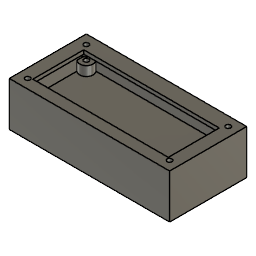
1602L_display_case (Autodesk Fusion 360 design; units mm, degrees)
Autodesk Fusion 360 part; units mm, degrees
sketch "Sketch1" plane through (0, 0, 0) normal (0, 0, 1) x (1, 0, 0)
  line L0 (0, 0) -> (80, 0)
  line L1 (80, 0) -> (80, 36)
  line L2 (80, 36) -> (0, 36)
  line L3 (0, 36) -> (0, 0)
  line L4 (-2.4, -2.4) -> (82.4, -2.4)
  line L5 (82.4, -2.4) -> (82.4, 38.4)
  line L6 (82.4, 38.4) -> (-2.4, 38.4)
  line L7 (-2.4, 38.4) -> (-2.4, -2.4)
  circle A0 centre (2.5, 33.5) radius 1.3
  circle A1 centre (2.5, 2.5) radius 1.3
  circle A2 centre (77.5, 2.5) radius 1.3
  circle A3 centre (77.5, 33.5) radius 1.3
  line L8 (4.2, 30.4) -> (75.8, 30.4)
  line L9 (75.8, 30.4) -> (75.8, 3.5)
  line L10 (75.8, 3.5) -> (4.2, 3.5)
  line L11 (4.2, 3.5) -> (4.2, 30.4)
  circle A4 centre (2.5, 33.5) radius 3.5
  circle A5 centre (77.5, 33.5) radius 3.5
  line L12 (-0.4, -0.4) -> (80.4, -0.4)
  line L13 (80.4, -0.4) -> (80.4, 36.4)
  line L14 (80.4, 36.4) -> (-0.4, 36.4)
  line L15 (-0.4, 36.4) -> (-0.4, -0.4)
  line L16 (-0.4, 6) -> (4.2, 6)
  line L17 (6, 3.5) -> (6, -0.4)
  line L18 (75.8, 6) -> (80.4, 6)
  line L19 (74, 3.5) -> (74, -0.4)
  circle A6 centre (2.5, 2.5) radius 3.5
  circle A7 centre (77.5, 2.5) radius 3.5
  point P0 (8, 33.5)
  dimension "d1" = 80
  dimension "d2" = 36
  dimension "d4" = 2.6
  dimension "d5" = 2.6
  dimension "d6" = 2.6
  dimension "d7" = 2.6
  dimension "d8" = 2.5
  dimension "d9" = 2.5
  dimension "d10" = 2.5
  dimension "d11" = 2.5
  dimension "d12" = 2.5
  dimension "d13" = 2.5
  dimension "d14" = 2.5
  dimension "d15" = 2.5
  dimension "d16" = 2.5
  dimension "d17" = 8
  dimension "d18" = 5.6
  dimension "d19" = 3.5
  dimension "d20" = 4.2
  dimension "d21" = 4.2
  dimension "d22" = 7
  dimension "d23" = 7
  dimension "d45" = 0.4
  dimension "d46" = 2
  dimension "d51" = 3.5
  dimension "d52" = 3.5
  dimension "d53" = 3.5
  dimension "d54" = 3.5
  dimension "d55" = 7
  dimension "d56" = 7
  constraint horizontal L0
  constraint vertical L1
  constraint horizontal L2
  constraint vertical L3
  constraint coincident L0.start L3.end
  constraint horizontal L8
  constraint vertical L9
  constraint horizontal L10
  constraint vertical L11
  constraint concentric A0 A4
  constraint concentric A3 A5
  constraint coincident L15 L16.start
  constraint coincident L11 L16.end
  constraint perpendicular L11 L16
  constraint coincident L10 L17.start
  constraint coincident L12 L17.end
  constraint perpendicular L12 L17
  constraint coincident L9 L18.start
  constraint coincident L13 L18.end
  constraint perpendicular L13 L18
  constraint coincident L10 L19.start
  constraint coincident L12 L19.end
  constraint perpendicular L12 L19
  constraint concentric A1 A6
  constraint concentric A2 A7
  measures "d1" distance of L0.start L0.end
  measures "d2" distance of L0.start L2.end
  measures "d4" diameter of A0
  measures "d5" diameter of A1
  measures "d6" diameter of A2
  measures "d7" diameter of A3
  measures "d8" distance of L2 A0.centre
  measures "d9" distance of L0 A1.centre
  measures "d10" distance of L0 A2.centre
  measures "d11" distance of L2 A3.centre
  measures "d12" distance of L3 A0.centre
  measures "d13" distance of L3 A1.centre
  measures "d14" distance of L1 A2.centre
  measures "d15" distance of L1 A3.centre
  measures "d16" distance of L2 P0
  measures "d17" distance of L3 P0
  measures "d18" distance of L2 L8
  measures "d19" distance of L0 L10
  measures "d20" distance of L3 L11
  measures "d21" distance of L1 L9
  measures "d22" diameter of A4
  measures "d23" diameter of A5
  measures "d46" distance of L6 L14
  measures "d51" distance of A1.centre L16
  measures "d52" distance of A1.centre L17
  measures "d53" distance of A2.centre L18
  measures "d54" distance of A2.centre L19
  measures "d55" diameter of A6
  measures "d56" diameter of A7
extrude "Extrude1" add sketch "Sketch1" along normal blind 7.2 contours L0 L3 A6 | L0 L3 L12 L15 A6 | L0 L3 L10 L11 A6 | L0 L12 A6 | L3 L15 A6 | L0 L17 A6 | L0 L12 L17 A6 | L12 A6 | L3 L15 L16 A6 | L3 L16 A6 | L15 A6 | L0 L10 L17 L19 | L0 L12 L17 L19 | L10 L17 A6 | L3 A4 L15 L16 | L1 L2 L3 L8 L9 L11 A4 A5 L16 L18 | L11 L16 A6 | L0 L19 A7 | L0 L12 L19 A7 | L3 A4 L15 | L2 L3 A4 | L0 L1 L9 L10 A7 | L0 L12 A7 | L10 L19 A7 | L2 L3 A4 L14 L15 | L2 L3 A4 | A4 L15 | L0 L1 A7 | L0 L1 L12 L13 A7 | L12 A7 | L2 A4 L14 | L2 A4 A5 L14 | L1 L13 A7 | L9 L18 A7 | A4 L14 | L2 A5 L14 | L1 L2 A5 | L1 L18 A7 | L1 L13 L18 A7 | L13 A7 | L1 L2 A5 L13 L14 | L1 L2 A5 | A5 L14 | L1 A5 L13 L18 | L1 A5 L13 | A5 L13 | L4 L5 L6 L7 makes body 1
extrude "Extrude2" cut sketch "Sketch1" along normal blind 5.2 contours L0 L10 L17 L19 | L0 L12 L17 L19 | L3 A4 L15 L16 | L1 L2 L3 L8 L9 L11 A4 A5 L16 L18 | L2 L3 A4 L14 L15 | L2 L3 A4 | L2 A4 A5 L14 | L1 L2 A5 L13 L14 | L1 L2 A5 | L1 A5 L13 L18 picked at (0.0168, 35.9832) picked at (79.9832, 35.9832) bodies 1
extrude "Extrude3" cut sketch "Sketch1" along normal blind 4 contours L0 L3 L10 L11 A6 | L3 L15 A6 | L12 L15 A6 | L0 L12 A6 | L0 L17 A6 | L0 L12 L17 A6 | L3 L15 L16 A6 | L3 L16 A6 | L10 L17 A6 | L11 L16 A6 | L0 L19 A7 | L0 L12 L19 A7 | L3 A4 L15 | L2 L3 A4 | L0 L1 L9 L10 A7 | L0 L12 A7 | L10 L19 A7 | L2 A4 L14 | L12 L13 A7 | L1 L13 A7 | L1 L18 A7 | L1 L13 L18 A7 | L9 L18 A7 | L2 A5 L14 | L1 L2 A5 | L1 A5 L13 bodies 1
extrude "Extrude4" add sketch "Sketch1" against normal blind 16.2 contours L12 A6 | L15 A6 | A4 L15 | L12 A7 | A4 L14 | L13 A7 | A5 L14 | A5 L13 | L4 L5 L6 L7 bodies 1
sketch "Sketch2" plane through (-2.4, 0, 0) normal (-1, 0, 0) x (0, -1, 0)
  line L0 (2.4, -16.2) -> (2.4, 7.2)
  line L1 (2.4, 7.2) -> (-38.4, 7.2)
  line L2 (-38.4, 7.2) -> (-38.4, -16.2)
  line L3 (-24.5, -6.6) -> (-11.5, -6.6)
  line L4 (-11.5, -6.6) -> (-11.5, -14.6)
  line L5 (-11.5, -14.6) -> (-24.5, -14.6)
  line L6 (-24.5, -14.6) -> (-24.5, -6.6)
  line L7 (-38.4, 0) -> (2.4, 0)
  line L8 (-38.4, -16.2) -> (2.4, -16.2)
  dimension "d35" = 6.6
  dimension "d36" = 8
  dimension "d37" = 13.9
  dimension "d38" = 13.9
  constraint horizontal L3
  constraint vertical L4
  constraint horizontal L5
  constraint vertical L6
  measures "d35" distance of L3 L7
  measures "d36" distance of L3 L5
  measures "d37" distance of L2 L6
  measures "d38" distance of L0 L4
extrude "Extrude5" cut sketch "Sketch2" against normal blind 2 contours L3 L4 L5 L6 bodies 1
extrude "Extrude6" add sketch "Sketch1" against normal blind 7 separate body contours L0 L3 A6 | L0 L3 L10 L11 A6 | L0 L17 A6 | L3 L16 A6 | L0 L10 L17 L19 | L10 L17 A6 | L1 L2 L3 L8 L9 L11 A4 A5 L16 L18 | L11 L16 A6 | L0 L19 A7 | L8 L9 L10 L11 A6 A7 | L10 L11 A6 | L2 L3 A4 | L0 L1 L9 L10 A7 | L10 L19 A7 | L2 L3 A4 | L0 L1 A7 | L9 L10 A7 | L9 L18 A7 | L1 L2 A5 | L1 L18 A7 | L1 L2 A5 makes body 2
extrude "Extrude7" cut sketch "Sketch1" against normal blind 5 contours L0 L3 A6 | L0 L17 A6 | L3 L16 A6 | L0 L10 L17 L19 | L10 L17 A6 | L1 L2 L3 L8 L9 L11 A4 A5 L16 L18 | L11 L16 A6 | L0 L19 A7 | L8 L9 L10 L11 A6 A7 | L10 L19 A7 | L0 L1 A7 | L9 L18 A7 | L1 L18 A7 bodies 2
